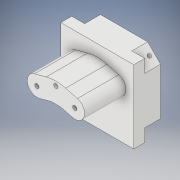
# Autodesk Inventor part: Base
Saved by Autodesk Inventor 2017 SP1 (Build 210196100, 196)
## iProperties
Created: 2018-02-11
Part Number: Base
Material: ABS Plastic
Document SubType Name: Modeling
Designer: Zach
Density: 1.06 g/cm^3
Appearance: CR White
Author: Zach
Autodesk Inventor part; units mm, degrees
ref_plane "YZ Plane" through (0, 0, 0) normal (1, 0, 0) x (0, 1, 0)
ref_plane "XZ Plane" through (0, 0, 0) normal (0, 1, 0) x (-1, 0, 0)
ref_plane "XY Plane" through (0, 0, 0) normal (0, 0, 1) x (1, 0, 0)
sketch "Sketch1" plane through (0, 0, 0) normal (0, 0, 1) x (1, 0, 0)
  line L0 (0, 0) -> (60, 0)
  line L1 (60, 0) -> (60, 60)
  line L2 (60, 60) -> (0, 60)
  line L3 (0, 60) -> (0, 0)
  dimension "d0" = 60
  dimension "d1" = 60
  constraints: 8 end point, 2 parallel, 1 horizontal, 1 perpendicular
  measures "d0" distance of L2.end L1.end
  measures "d1" distance of L1.end L0.end
extrude "Extrusion1" add sketch "Sketch1" along normal blind 22
sketch "Sketch2" plane through (0, 0, 0) normal (0, 0, -1) x (-1, 0, 0)
  line L0 (0, 10.6066) -> (-10.6066, 0)
  line L1 (0, 10.6066) -> (0, 0)
  line L2 (0, 0) -> (-10.6066, 0)
  line L3 (0, 60) -> (-10.6066, 60)
  line L4 (-10.6066, 60) -> (0, 49.3934)
  line L5 (0, 49.3934) -> (0, 60)
  line L6 (-49.3934, 60) -> (-60, 60)
  line L7 (-60, 60) -> (-60, 49.3934)
  line L8 (-49.3934, 60) -> (-60, 49.3934)
  line L9 (-49.3934, 0) -> (-60, 0)
  line L10 (-60, 0) -> (-60, 10.6066)
  line L11 (-49.3934, 0) -> (-60, 10.6066)
  dimension "d4" = 15
  dimension "d7" = 15
  dimension "d8" = 15
  dimension "d9" = 15
  constraints: 24 end point, 4 horizontal, 4 perpendicular, 4 vertical
  measures "d4" distance of L0.start L0.end
  measures "d7" distance of L3.end L4.end
  measures "d8" distance of L6.start L7.end
  measures "d9" distance of L9.start L10.end
extrude "Extrusion2" cut sketch "Sketch2" against normal blind 13
sketch "Sketch7" plane through (0, 0, 22) normal (0, 0, 1) x (1, 0, 0)
  circle A0 centre (45.5887, 39) radius 8 construction
  circle A1 centre (14.4113, 39) radius 8 construction
  line L0 (22, 49.3156) -> (26.1411, 33.8608) construction
  line L1 (26.1411, 33.8608) -> (16.4818, 31.2726)
  line L2 (12.3407, 46.7274) -> (22, 49.3156)
  line L3 (33.8589, 33.8608) -> (38, 49.3156) construction
  line L4 (38, 49.3156) -> (47.6593, 46.7274)
  line L5 (33.8589, 33.8608) -> (43.5182, 31.2726)
  line L6 (22, 49.3156) -> (38, 49.3156) construction
  line L7 (26.1411, 33.8608) -> (33.8589, 33.8608)
  arc A2 (12.3407, 46.7274) -> (16.4818, 31.2726) centre (14.4113, 39) ccw
  arc A3 (43.5182, 31.2726) -> (47.6593, 46.7274) centre (45.5887, 39) ccw
  line L8 (60, 60) -> (0, 60) projected
  arc A4 (38, 49.3156) -> (22, 49.3156) centre (30, 19.4592) ccw
  point P0 (0, 0)
  point P1 (30, 49.3156)
  point P2 (30, 60)
  dimension "d28" = 16
  dimension "d29" = 16
  dimension "d30" = 16
  dimension "d31" = 10
  dimension "d32" = 10
  dimension "d33" = 16
  dimension "d34" = 16
  dimension "d36" = 75
  dimension "d37" = 21
  constraints: 16 end point, 10 point on circle, 10 tangent, 5 centre point, 2 horizontal alignment, 2 midpoint, 2 perpendicular, 1 horizontal, 1 point on line, 1 vertical alignment
  measures "d28" diameter of A0
  measures "d29" diameter of A1
  measures "d30" distance of L0.start L0.end
  measures "d31" distance from line of A1.centre L0
  measures "d32" distance from line of L3 A0.centre
  measures "d33" distance of L3.start L3.end
  measures "d34" distance of L0.start L3.end
  measures "d36" angle of L6 L0
  measures "d37" distance from line of L8 A2.centre
extrude "Extrusion7" add sketch "Sketch7" along normal blind 34
sketch "Sketch8" plane through (10.6066, 0, 13) normal (-0.7071, -0.7071, 0) x (-0.7071, 0.7071, 0)
  circle A0 centre (7.5, 9) radius 1.5
  line L0 (0, 13) -> (15, 13) projected
  point P0 (7.5, 13)
  point P1 (7.5, 13)
  dimension "d40" = 3
  dimension "d41" = 4
  constraints: 1 centre point, 1 midpoint, 1 vertical alignment
  measures "d40" diameter of A0
  measures "d41" distance of point (7.5, 13) A0.centre
extrude "Extrusion8" cut sketch "Sketch8" against normal through all
sketch "Sketch9" plane through (60, 10.6066, 13) normal (0.7071, -0.7071, 0) x (-0.7071, -0.7071, 0)
  circle A0 centre (7.5, 9) radius 1.5
  line L0 (0, 13) -> (15, 13) projected
  point P0 (49.9264, 13)
  point P1 (7.5, 13)
  dimension "d44" = 3
  dimension "d45" = 4
  constraints: 1 centre point, 1 midpoint, 1 vertical alignment
  measures "d44" diameter of A0
  measures "d45" distance of point (7.5, 13) A0.centre
extrude "Extrusion9" cut sketch "Sketch9" against normal through all
sketch "Sketch10" plane through (0, 0, 56) normal (0, 0, 1) x (1, 0, 0)
  line L0 (22, 49.3156) -> (12.3407, 46.7274) construction
  arc A0 (12.3407, 46.7274) -> (16.4818, 31.2726) centre (14.4113, 39) ccw construction
  line L1 (16.4818, 31.2726) -> (26.1411, 33.8608) construction
  line L2 (26.1411, 33.8608) -> (33.8589, 33.8608) construction
  line L3 (33.8589, 33.8608) -> (43.5182, 31.2726) construction
  arc A1 (43.5182, 31.2726) -> (47.6593, 46.7274) centre (45.5887, 39) ccw construction
  line L4 (47.6593, 46.7274) -> (38, 49.3156) construction
  arc A2 (38, 49.3156) -> (22, 49.3156) centre (30, 19.4592) ccw construction
  circle A3 centre (14.4113, 39) radius 1.75
  circle A4 centre (45.5887, 39) radius 1.75
  circle A5 centre (30, 46.8608) radius 1.75
  point P0 (0, 0)
  point P1 (30, 33.8608)
  dimension "d48" = 3.5
  dimension "d49" = 3.5
  dimension "d50" = 3.5
  dimension "d51" = 13
  constraints: 3 centre point, 2 coincident, 1 midpoint, 1 vertical alignment
  measures "d48" diameter of A3
  measures "d49" diameter of A4
  measures "d50" diameter of A5
  measures "d51" distance from line of L2 A5.centre
extrude "Extrusion10" cut sketch "Sketch10" against normal blind 29
body "Solid1"
